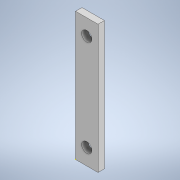
# Autodesk Inventor part: リンク
Saved by Autodesk Inventor 2021 (Build 250183000, 183)
## iProperties
Created: 2021-10-09
Part Number: リンク
Material: 一般
Document SubType Name: Modeling
Designer: ryusei
Density: 1 g/cm^3
Appearance: 既定
Author: ryusei
Autodesk Inventor part; units mm, degrees
ref_plane "YZ Plane" through (0, 0, 0) normal (1, 0, 0) x (0, 1, 0)
ref_plane "XZ Plane" through (0, 0, 0) normal (0, 1, 0) x (-1, 0, 0)
ref_plane "XY Plane" through (0, 0, 0) normal (0, 0, 1) x (1, 0, 0)
sketch "スケッチ1" plane through (0, 0, 0) normal (0, 0, 1) x (1, 0, 0)
  line L0 (0, 0) -> (7, 0)
  line L1 (7, 0) -> (7, 40)
  line L2 (7, 40) -> (0, 40)
  line L3 (0, 40) -> (0, 0)
  dimension "d0" = 7
  dimension "d1" = 40
  constraints: 8 end point, 2 parallel, 1 horizontal, 1 perpendicular
  measures "d0" distance of L0.start L0.end
  measures "d1" distance of L0.end L1.end
extrude "押し出し1" add sketch "スケッチ1" along normal blind 2
sketch "スケッチ2" plane through (0, 0, 2) normal (0, 0, 1) x (1, 0, 0)
  line L0 (7, 0) -> (7, 40) projected
  line L1 (7, 40) -> (0, 40) projected
  line L2 (0, 0) -> (7, 0) projected
  point P0 (3.5, 35)
  point P1 (3.5, 5)
  dimension "d4" = 3.5
  dimension "d5" = 5
  dimension "d6" = 3.5
  dimension "d7" = 5
  measures "d4" distance from line of L0 point (3.5, 35)
  measures "d5" distance from line of point (3.5, 35) L1
  measures "d6" distance from line of L0 point (3.5, 5)
  measures "d7" distance from line of L2 point (3.5, 5)
hole "穴1" at (3.5, 35, 2) at (3.5, 5, 2) direction (0, 0, -1) diameter 3.2 end through all
sketch "スケッチ3" plane through (0, 0, 2) normal (0, 0, 1) x (1, 0, 0)
  point P0 (0, 0)
